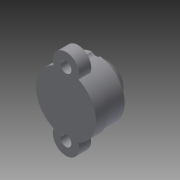
# Autodesk Inventor part: BallCaster
Saved by Autodesk Inventor 2015 (Build 190159000, 159)
## iProperties
Created: 2015-04-05
Part Number: BallCaster
Material: Generic
Document SubType Name: Modeling
Designer: Jesse
Density: 1 g/cm^3
Appearance: Default
Author: Jesse
Autodesk Inventor part; units mm, degrees
ref_plane "YZ Plane" through (0, 0, 0) normal (1, 0, 0) x (0, 1, 0)
ref_plane "XZ Plane" through (0, 0, 0) normal (0, 1, 0) x (-1, 0, 0)
ref_plane "XY Plane" through (0, 0, 0) normal (0, 0, 1) x (1, 0, 0)
sketch "Sketch1" plane through (0, 0, 0) normal (0, 1, 0) x (-1, 0, 0)
  circle A0 centre (0, 0) radius 6.35
  circle A1 centre (0.0105, -6.731) radius 1.143
  circle A2 centre (-0.0105, 6.731) radius 1.143
  circle A3 centre (-0.0105, 6.731) radius 2.8045
  circle A4 centre (0.0105, -6.731) radius 2.7835
  line L0 (2.794, 10.5755) -> (2.794, -14.4258)
  line L1 (4.742, 9.5355) -> (-5.3201, 9.5355)
  line L2 (6.3395, -9.5145) -> (-5.3201, -9.5145)
  arc A5 (-1.0529, 6.2621) -> (1.0333, 6.2654) centre (-0.0105, 6.731) ccw
  arc A6 (1.0529, -6.2621) -> (-1.0333, -6.2654) centre (0.0105, -6.731) ccw
  dimension "d0" = 12.7
  dimension "d1" = 2.286
  dimension "d2" = 2.286
  dimension "d3" = 6.731
  dimension "d4" = 6.731
  dimension "d5" = 13.462
  dimension "d6" = 19.05
  constraints: 12 point on circle, 7 centre point, 6 end point, 4 tangent, 3 coincident, 2 concentric, 2 horizontal, 1 vertical
  measures "d0" diameter of A0
  measures "d1" diameter of A1
  measures "d2" diameter of A2
  measures "d3" distance of point (0, 0) A2.centre
  measures "d4" distance of point (0, 0) A1.centre
  measures "d5" distance of A2.centre A1.centre
  measures "d6" distance between parallel lines of L2 L1
extrude "Extrusion1" add sketch "Sketch1" along normal blind 2.54 contours A2 A0 A3 | A0 A3 A2 | A0 L0 A4 A3 | A0 L0 | A4 A0 A1 | A0 A1 A4
sketch "Sketch2" plane through (0, 2.54, 0) normal (0, 1, 0) x (1, 0, 0)
  circle A0 centre (0, 0) radius 6.0643
  circle A1 centre (0, 0) radius 5.2578
  circle A2 centre (-0.0105, 6.731) radius 1.143 projected
  arc A3 (0.8695, 6.0016) -> (-0.8883, 5.9988) centre (0, 0) ccw
  arc A4 (-0.8555, -6.0036) -> (0.8879, -5.9989) centre (0, 0) ccw
  arc A5 (0.8879, -5.9989) -> (-0.8555, -6.0036) centre (0.0181, -6.7139) ccw
  arc A6 (-0.8883, 5.9988) -> (0.8695, 6.0016) centre (-0.0105, 6.731) ccw
  line L0 (0, 0) -> (0.8695, 0)
  line L1 (0.8695, 0) -> (0.8695, 1.0578)
  line L2 (0.8695, 1.0578) -> (0, 1.0578)
  line L3 (0, 1.0578) -> (0, 0)
  constraints: 16 point on circle, 8 end point, 6 centre point, 2 coincident, 2 concentric, 2 parallel, 1 horizontal, 1 perpendicular
extrude "Extrusion2" add sketch "Sketch2" along normal blind 3.81 contours A0 A5 A2 | L3 L2 L1 L0
sketch "Sketch3" plane through (0, 2.54, -1.0578) normal (-1, 0, 0) x (0, 0, 1)
  circle A0 centre (1.0578, 2.54) radius 5.08
  line L0 (1.0578, 7.62) -> (7.9844, 7.62)
  line L1 (6.8385, -2.54) -> (-4.7233, -2.54) projected
  line L2 (1.0578, 7.62) -> (1.0578, 0)
  line L3 (1.0578, 7.62) -> (1.0578, -2.54)
  dimension "d11" = 10.16
  dimension "d12" = 10.16
  constraints: 6 end point, 2 point on circle, 1 centre point, 1 horizontal, 1 point on line, 1 tangent, 1 vertical
  measures "d11" diameter of A0
  measures "d12" distance between parallel lines of L0 L1
revolve "Revolution1" add sketch "Sketch3" angle 360 about axis through (0, 10.16, 0) along (0, -1, 0) picked at (1.4346, 5.0375) contours A0 L3 L2
body "Solid1"
